Turret Base Top Plate_v10 (Autodesk Fusion 360 design; units mm, degrees)
Autodesk Fusion 360 part; units mm, degrees
sketch "Sketch1" plane through (0, 0, 0) normal (1, 0, 0) x (0, 1, 0)
  line L0 (36.1, 2.8393) -> (36.1, 0.1999) construction
  line L1 (29.9076, 4.5417) -> (29.928, 4.4966)
  line L2 (-31.8, -5.5) -> (-31.8, -3.2628) construction
  line L3 (-36.1, 2.8393) -> (-36.1, 0.1999) construction
  line L4 (30.0626, 4.563) -> (30.0813, 4.5279) construction
  line L5 (31.4586, -3.1214) -> (30.1778, -4.4022) construction
  arc A0 (-31.3525, -3.0154) -> (-31.95, -3.2628) centre (-31.6, -3.2628) ccw
  line L6 (30.0462, 4.5991) -> (30.0626, 4.563) construction
  line L7 (30.1023, 4.4942) -> (30.1254, 4.4619) construction
  arc A1 (31.8, -3.2628) -> (31.4586, -3.1214) centre (31.6, -3.2628) ccw construction
  line L8 (30.0322, 4.6363) -> (30.0462, 4.5991) construction
  line L9 (31.8, -5.5) -> (31.8, -3.2628) construction
  line L10 (-31.95, -5.35) -> (-31.95, -3.2628)
  line L11 (-31.8, -5.5) -> (-31.8, -3.2628) construction
  line L12 (35.15, 10) -> (31.5, 10) construction
  line L13 (29.9514, 4.4529) -> (29.9775, 4.4108)
  arc A2 (-31.4586, -3.1214) -> (-31.8, -3.2628) centre (-31.6, -3.2628) ccw construction
  line L14 (31.95, -5.35) -> (31.95, -3.2628)
  line L15 (-33.4393, -5.5) -> (-31.8, -5.5) construction
  line L16 (33.4393, -5.5) -> (31.8, -5.5) construction
  line L17 (31.3525, -3.0154) -> (30.3679, -4)
  line L18 (29.8757, 4.6355) -> (29.8901, 4.5881)
  line L19 (29.8901, 4.5881) -> (29.9076, 4.5417)
  line L20 (-33.4393, -5.5) -> (-31.8, -5.5) construction
  arc A3 (-31.4586, -3.1214) -> (-31.8, -3.2628) centre (-31.6, -3.2628) ccw construction
  line L21 (35.15, 10) -> (31.5, 10) construction
  line L22 (-33.3772, -5.35) -> (-31.95, -5.35)
  line L23 (33.3772, 5.35) -> (35.95, 2.7772)
  line L24 (36.1, 2.8393) -> (36.1, 0.1999) construction
  line L25 (-31.3525, -3.0154) -> (-30.3679, -4)
  arc A4 (31.95, -3.2628) -> (31.3525, -3.0154) centre (31.6, -3.2628) ccw
  line L26 (33.4393, -5.5) -> (31.8, -5.5) construction
  line L27 (35.95, 2.7772) -> (35.95, 0.1377)
  arc A5 (31.8, -3.2628) -> (31.4586, -3.1214) centre (31.6, -3.2628) ccw construction
  line L28 (31.4586, -3.1214) -> (30.1778, -4.4022) construction
  line L29 (33.3772, -5.35) -> (31.95, -5.35)
  line L30 (31.8, -5.5) -> (31.8, -3.2628) construction
  line L31 (-29.9076, 4.5417) -> (-29.928, 4.4966)
  line L32 (-30.0626, 4.563) -> (-30.0813, 4.5279) construction
  line L33 (-36.1, 0.1999) -> (-36.2999, 0) construction
  line L34 (-30.0064, 4.3705) -> (-30.0378, 4.3322)
  line L35 (36.1, -0.1999) -> (36.1, -2.8393) construction
  line L36 (-30.1023, 4.4942) -> (-30.1254, 4.4619) construction
  line L37 (-30.0813, 4.5279) -> (-30.1023, 4.4942) construction
  line L38 (35.95, -0.1377) -> (35.95, -2.7772)
  line L39 (-29.8901, 4.5881) -> (-29.9076, 4.5417)
  line L40 (30.0117, 4.713) -> (30.0207, 4.6743) construction
  line L41 (-36.1, -0.1999) -> (-36.1, -2.8393) construction
  circle A6 centre (-40, 0) radius 2.1 construction
  line L42 (-30.0462, 4.5991) -> (-30.0626, 4.563) construction
  line L43 (30.0052, 4.7522) -> (30.0117, 4.713) construction
  line L44 (30.1023, 4.4942) -> (30.1254, 4.4619) construction
  line L45 (-30.0462, 4.5991) -> (-30.0626, 4.563) construction
  line L46 (30.0462, 4.5991) -> (30.0626, 4.563) construction
  line L47 (30.1254, 4.4619) -> (30.1506, 4.4312) construction
  line L48 (-36.1, 0.1999) -> (-36.2999, 0) construction
  line L49 (30.0813, 4.5279) -> (30.1023, 4.4942) construction
  line L50 (30.0626, 4.563) -> (30.0813, 4.5279) construction
  line L51 (-30.0813, 4.5279) -> (-30.1023, 4.4942) construction
  line L52 (29.9775, 4.4108) -> (30.0064, 4.3705)
  line L53 (-30.0626, 4.563) -> (-30.0813, 4.5279) construction
  line L54 (-36.2999, 0) -> (-36.1, -0.1999) construction
  line L55 (30.0378, 4.3322) -> (30.07, 4.2979)
  line L56 (30.0322, 4.6363) -> (30.0462, 4.5991) construction
  line L57 (30.0064, 4.3705) -> (30.0378, 4.3322)
  line L58 (-29.9775, 4.4108) -> (-30.0064, 4.3705)
  line L59 (-36.1, -0.1999) -> (-36.1, -2.8393) construction
  line L60 (-35.95, -0.1377) -> (-35.95, -2.7772)
  line L61 (-30.0378, 4.3322) -> (-30.07, 4.2979)
  line L62 (-36.2999, 0) -> (-36.1, -0.1999) construction
  line L63 (30.0813, 4.5279) -> (30.1023, 4.4942) construction
  line L64 (29.928, 4.4966) -> (29.9514, 4.4529)
  line L65 (-30.1254, 4.4619) -> (-30.1506, 4.4312) construction
  line L66 (-30.1254, 4.4619) -> (-30.1506, 4.4312) construction
  line L67 (30.1254, 4.4619) -> (30.1506, 4.4312) construction
  line L68 (-30.1023, 4.4942) -> (-30.1254, 4.4619) construction
  line L69 (36.1, 0.1999) -> (36.2999, 0) construction
  line L70 (-29.9514, 4.4529) -> (-29.9775, 4.4108)
  line L71 (30.0117, 4.713) -> (30.0207, 4.6743) construction
  line L72 (-29.928, 4.4966) -> (-29.9514, 4.4529)
  line L73 (29.8564, 4.7326) -> (29.8645, 4.6837)
  line L74 (30.0013, 4.7917) -> (30.0052, 4.7522) construction
  line L75 (-30.0322, 4.6363) -> (-30.0462, 4.5991) construction
  line L76 (-29.8757, 4.6355) -> (-29.8901, 4.5881)
  line L77 (30.07, 4.2979) -> (31.3525, 3.0154)
  line L78 (36.1, -0.1999) -> (36.1, -2.8393) construction
  circle A7 centre (40, 0) radius 2.1 construction
  line L79 (30.1506, 4.4312) -> (30.1778, 4.4022) construction
  circle A8 centre (40, 0) radius 2.1 construction
  line L80 (-35.15, 10) -> (-31.5, 10) construction
  line L81 (-30.0207, 4.6743) -> (-30.0322, 4.6363) construction
  line L82 (30.1506, 4.4312) -> (30.1778, 4.4022) construction
  line L83 (-29.8515, 4.7819) -> (-29.8564, 4.7326)
  line L84 (-30.0052, 4.7522) -> (-30.0117, 4.713) construction
  line L85 (-29.8645, 4.6837) -> (-29.8757, 4.6355)
  line L86 (36.1, 0.1999) -> (36.2999, 0) construction
  line L87 (-35, 10.15) -> (-31.5, 10.15)
  line L88 (36.2999, 0) -> (36.1, -0.1999) construction
  line L89 (30.0207, 4.6743) -> (30.0322, 4.6363) construction
  line L90 (-30.0052, 4.7522) -> (-30.0117, 4.713) construction
  line L91 (30.0207, 4.6743) -> (30.0322, 4.6363) construction
  line L92 (29.8645, 4.6837) -> (29.8757, 4.6355)
  line L93 (-35.95, -2.7772) -> (-33.3772, -5.35)
  line L94 (-36.1, -2.8393) -> (-33.4393, -5.5) construction
  line L95 (30.0013, 4.7917) -> (30.0052, 4.7522) construction
  line L96 (33.4393, 5.5) -> (36.1, 2.8393) construction
  line L97 (-30.0013, 4.7917) -> (-30.0052, 4.7522) construction
  line L98 (-30.0013, 4.7917) -> (-30.0052, 4.7522) construction
  line L99 (-30.0117, 4.713) -> (-30.0207, 4.6743) construction
  line L100 (30.1778, 4.4022) -> (31.4586, 3.1214) construction
  line L101 (30.0052, 4.7522) -> (30.0117, 4.713) construction
  line L102 (36.1, -2.8393) -> (33.4393, -5.5) construction
  line L103 (30.1778, 4.4022) -> (31.4586, 3.1214) construction
  line L104 (-30.0117, 4.713) -> (-30.0207, 4.6743) construction
  line L105 (-33.4393, 5.5) -> (-36.1, 2.8393) construction
  line L106 (-29.8564, 4.7326) -> (-29.8645, 4.6837)
  line L107 (36.1, -2.8393) -> (33.4393, -5.5) construction
  line L108 (-33.3772, 5.35) -> (-35.95, 2.7772)
  arc A9 (31.4586, 3.1214) -> (31.8, 3.2628) centre (31.6, 3.2628) ccw construction
  line L109 (29.8515, 4.7819) -> (29.8564, 4.7326)
  line L110 (36.2999, 0) -> (36.1, -0.1999) construction
  line L111 (-36.1, -2.8393) -> (-33.4393, -5.5) construction
  line L112 (-30.0207, 4.6743) -> (-30.0322, 4.6363) construction
  arc A10 (31.4586, 3.1214) -> (31.8, 3.2628) centre (31.6, 3.2628) ccw construction
  arc A11 (31.3525, 3.0154) -> (31.95, 3.2628) centre (31.6, 3.2628) ccw
  line L113 (35.95, -2.7772) -> (33.3772, -5.35)
  line L114 (33.4393, 5.5) -> (36.1, 2.8393) construction
  line L115 (35, 10.15) -> (31.5, 10.15)
  circle A12 centre (-40, 0) radius 2.1 construction
  line L116 (-30.0322, 4.6363) -> (-30.0462, 4.5991) construction
  line L117 (-31.95, 5.35) -> (-33.3772, 5.35)
  line L118 (30, 4.8314) -> (30.0013, 4.7917) construction
  line L119 (29.85, 4.829) -> (29.8515, 4.7819)
  line L120 (-30.1778, 4.4022) -> (-31.4586, 3.1214) construction
  line L121 (31.8, 5.5) -> (33.4393, 5.5) construction
  line L122 (-35.2083, 9.9987) -> (-35.15, 10) construction
  line L123 (-30, 4.8314) -> (-30.0013, 4.7917) construction
  line L124 (-35.2083, 9.9987) -> (-35.15, 10) construction
  arc A13 (30.5, 10) -> (30, 9.5) centre (30.5, 9.5) ccw construction
  line L125 (-31.95, 3.2628) -> (-31.95, 5.35)
  line L126 (-29.85, 4.829) -> (-29.8515, 4.7819)
  line L127 (30, 9.5) -> (30, 8.5) construction
  arc A14 (30.5, 10.15) -> (29.85, 9.5) centre (30.5, 9.5) ccw
  line L128 (30, 9.5) -> (30, 8.5) construction
  line L129 (31.95, 3.2628) -> (31.95, 5.35)
  arc A15 (-31.8, 3.2628) -> (-31.4586, 3.1214) centre (-31.6, 3.2628) ccw construction
  arc A16 (-31.8, 3.2628) -> (-31.4586, 3.1214) centre (-31.6, 3.2628) ccw construction
  line L130 (31.95, 5.35) -> (33.3772, 5.35)
  line L131 (-30.07, 4.2979) -> (-31.3525, 3.0154)
  arc A17 (-31.95, 3.2628) -> (-31.3525, 3.0154) centre (-31.6, 3.2628) ccw
  line L132 (-33.4393, 5.5) -> (-36.1, 2.8393) construction
  line L133 (-30.1506, 4.4312) -> (-30.1778, 4.4022) construction
  line L134 (29.85, 9.5) -> (29.85, 8.5)
  line L135 (-30.1778, 4.4022) -> (-31.4586, 3.1214) construction
  line L136 (31.5, 10) -> (30.5, 10) construction
  line L137 (30, 8.5) -> (30, 4.8314) construction
  line L138 (-31.5, 10) -> (-30.5, 10) construction
  line L139 (31.8, 3.2628) -> (31.8, 5.5) construction
  line L140 (30, 4.8314) -> (30.0013, 4.7917) construction
  line L141 (-31.5, 10.15) -> (-30.5, 10.15)
  arc A18 (30.5, 10) -> (30, 9.5) centre (30.5, 9.5) ccw construction
  arc A19 (-30, 9.5) -> (-30.5, 10) centre (-30.5, 9.5) ccw construction
  line L142 (-30.1506, 4.4312) -> (-30.1778, 4.4022) construction
  line L143 (31.8, 5.5) -> (33.4393, 5.5) construction
  line L144 (-35.15, 10) -> (-31.5, 10) construction
  line L145 (31.8, 3.2628) -> (31.8, 5.5) construction
  line L146 (30, 8.5) -> (30, 4.8314) construction
  line L147 (-30, 4.8314) -> (-30.0013, 4.7917) construction
  line L148 (29.85, 8.5) -> (29.85, 4.829)
  line L149 (-30, 9.5) -> (-30, 8.5) construction
  line L150 (-29.85, 9.5) -> (-29.85, 8.5)
  arc A20 (-29.85, 9.5) -> (-30.5, 10.15) centre (-30.5, 9.5) ccw
  line L151 (31.5, 10) -> (30.5, 10) construction
  line L152 (-29.85, 8.5) -> (-29.85, 4.829)
  line L153 (-31.8, 5.5) -> (-33.4393, 5.5) construction
  line L154 (-31.8, 3.2628) -> (-31.8, 5.5) construction
  arc A21 (-30, 9.5) -> (-30.5, 10) centre (-30.5, 9.5) ccw construction
  line L155 (-31.8, 5.5) -> (-33.4393, 5.5) construction
  line L156 (-31.5, 10) -> (-30.5, 10) construction
  line L157 (-31.8, 3.2628) -> (-31.8, 5.5) construction
  line L158 (-30, 9.5) -> (-30, 8.5) construction
  line L159 (-30, 8.5) -> (-30, 4.8314) construction
  line L160 (31.5, 10.15) -> (30.5, 10.15)
  line L161 (-30, 8.5) -> (-30, 4.8314) construction
  line L162 (0, 15) -> (0, -15) construction
  line L163 (-35.95, 2.7772) -> (-35.95, 0.1377)
  line L164 (-36.1, 2.8393) -> (-36.1, 0.1999) construction
  line L165 (35, 10.15) -> (35, 12)
  line L166 (35, 12) -> (-35, 12)
  line L167 (-35, 12) -> (-35, 10.15)
  line L168 (30.3679, -4) -> (27.5, -4)
  line L169 (27.5, -4) -> (27.5, 9.5)
  line L170 (27.5, 9.5) -> (-27.5, 9.5)
  line L171 (-27.5, 9.5) -> (-27.5, -4)
  line L172 (-27.5, -4) -> (-30.3679, -4)
  line L173 (35.95, 0.1377) -> (35.95, -0.1377)
  line L174 (-35.95, 0.1377) -> (-35.95, -0.1377)
  dimension "d1" = 16
  constraint vertical L162
  constraint parallel L12 L115
  constraint parallel L151 L160
  constraint concentric A13 A14
  constraint parallel L128 L134
  constraint parallel L137 L148
  constraint parallel L119 L140
  constraint parallel L95 L109
  constraint parallel L73 L101
  constraint parallel L71 L92
  constraint parallel L18 L91
  constraint parallel L8 L19
  constraint parallel L1 L46
  constraint parallel L50 L64
  constraint parallel L13 L63
  constraint parallel L44 L52
  constraint parallel L47 L57
  constraint parallel L55 L79
  constraint parallel L77 L103
  constraint concentric A10 A11
  constraint parallel L129 L145
  constraint parallel L130 L143
  constraint parallel L23 L96
  constraint parallel L24 L27
  constraint parallel L35 L38
  constraint parallel L102 L113
  constraint parallel L26 L29
  constraint parallel L14 L30
  constraint concentric A1 A4
  constraint parallel L5 L17
  constraint tangent L17 A4
  constraint tangent A14 L160
  constraint tangent A14 L134
  constraint tangent L77 A11
  constraint tangent A11 L129
  constraint tangent L14 A4
  constraint symmetric L47.end L65.end L162
  constraint symmetric A13.start L138.end L162
  constraint symmetric L8.start L75.start L162
  constraint symmetric L4.start L32.start L162
  constraint symmetric L6.start L42.start L162
  constraint symmetric L40.end L81.start L162
  constraint symmetric L4.end L32.end L162
  constraint symmetric L127.end L149.end L162
  constraint symmetric L118.start L123.start L162
  constraint symmetric L74.start L97.start L162
  constraint symmetric L40.start L84.end L162
  constraint symmetric L7.start L36.start L162
  constraint symmetric A13.end A19.start L162
  constraint symmetric L43.start L84.start L162
  constraint symmetric L7.end L36.end L162
  constraint symmetric L79.end L120.start L162
  constraint symmetric L5.start A2.start L162
  constraint symmetric A9.end A15.start L162
  constraint symmetric L12.start L80.start L162
  constraint symmetric L12.end L80.end L162
  constraint symmetric L2.start L9.start L162
  constraint symmetric A1.start L2.end L162
  constraint symmetric L35.end L41.end L162
  constraint symmetric L15.start L16.start L162
  constraint symmetric L41.start L35.start L162
  constraint symmetric L96.start L105.start L162
  constraint symmetric L0.end L3.end L162
  constraint symmetric L121.start L153.start L162
  constraint symmetric L3.start L0.start L162
  constraint symmetric A15.start A9.end L162
  constraint symmetric L120.end L100.end L162
  constraint symmetric L35.start L41.start L162
  constraint symmetric L69.end L33.end L162
  constraint symmetric L105.start L96.start L162
  constraint symmetric A1 A2 L162
  constraint symmetric A3 A5 L162
  constraint symmetric A9 A15 L162
  constraint symmetric A6 A7 L162
  constraint symmetric A8 A12 L162
  constraint symmetric A13 A19 L162
  constraint symmetric A18 A21 L162
  constraint symmetric A10 A16 L162
  constraint symmetric L87.start L115.start L162
  constraint symmetric L87.end L115.end L162
  constraint symmetric L141.end A14.start L162
  constraint symmetric L150.start A14.end L162
  constraint symmetric A14 A20 L162
  constraint symmetric L150.end L134.end L162
  constraint symmetric L126.start L119.start L162
  constraint symmetric L83.start L109.start L162
  constraint symmetric L83.end L73.start L162
  constraint symmetric L85.start L73.end L162
  constraint symmetric L76.start L18.start L162
  constraint symmetric L39.start L18.end L162
  constraint symmetric L31.start L1.start L162
  constraint symmetric L31.end L1.end L162
  constraint symmetric L70.start L13.start L162
  constraint symmetric L58.start L13.end L162
  constraint symmetric L34.start L52.end L162
  constraint symmetric L34.end L55.start L162
  constraint symmetric L61.end L55.end L162
  constraint symmetric L131.end L77.end L162
  constraint symmetric L125.start A11.end L162
  constraint symmetric A11 A17 L162
  constraint symmetric L117.start L129.end L162
  constraint symmetric L108.start L23.start L162
  constraint symmetric L108.end L23.end L162
  constraint symmetric L163.end L27.end L162
  constraint symmetric L38.start L60.start L162
  constraint symmetric L38.end L60.end L162
  constraint symmetric L22.start L29.start L162
  constraint symmetric L10.start L14.start L162
  constraint symmetric L14.end A0.end L162
  constraint symmetric L17.start A0.start L162
  constraint symmetric A0 A4 L162
  constraint symmetric L17.end L25.end L162
  constraint horizontal L115
  constraint coincident L21.start L12
  constraint parallel L12 L21
  constraint perpendicular L115 L165
  constraint perpendicular L134 L166
  constraint horizontal L168
  constraint perpendicular L168 L169
  constraint perpendicular L169 L170
  constraint perpendicular L170 L171
  constraint perpendicular L171 L172
  constraint parallel L38 L173
  measures "d1" distance of L166 L172
extrude "Extrude1" add sketch "Sketch1" along normal blind 109
fillet "Fillet1" radius 5 2 edges at (54.5, -27.5, 9.5) (54.5, 27.5, 9.5)
sketch "Sketch2" plane through (0, 0, 12) normal (0, 0, 1) x (-1, 0, 0)
  line L0 (0, -35) -> (0, 35)
  line L1 (0, 35) -> (-109, 35)
  line L2 (-109, 35) -> (-109, -35)
  line L3 (-109, -35) -> (0, -35)
  line L4 (-109, 0) -> (0, 0) construction
  line L5 (-69, 0) -> (-89, 0) construction
  circle A0 centre (-89, 0) radius 8
  circle A1 centre (-79, -17.3205) radius 8
  circle A2 centre (-59, -17.3205) radius 8
  circle A3 centre (-49, 0) radius 8
  circle A4 centre (-59, 17.3205) radius 8
  circle A5 centre (-79, 17.3205) radius 8
  dimension "d11" = 20
  dimension "d12" = 16
  dimension "d14" = 360
  constraint midpoint L2 L4.start
  constraint coincident L4.end origin
  constraint coincident L4 L5.start
  constraint coincident L5.end A0.centre
  measures "d11" distance of L5.start L5.end
  measures "d12" diameter of A0
extrude "Extrude2" cut sketch "Sketch2" against normal blind 3 contours A0 | A1 | A2 | A3 | A4 | A5
